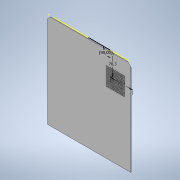
# Autodesk Inventor part: klapa
Saved by Autodesk Inventor 2020 (Build 240168000, 168)
## iProperties
Created: 2019-11-16
Part Number: klapa
Material: Ogólny
Document SubType Name: Modeling
Designer: Hubert Słomion
Density: 1 g/cm^3
Appearance: Domyślna
Author: Hubert Słomion
Autodesk Inventor part; units mm, degrees
ref_plane "YZ Plane" through (0, 0, 0) normal (1, 0, 0) x (0, 1, 0)
ref_plane "XZ Plane" through (0, 0, 0) normal (0, 1, 0) x (-1, 0, 0)
ref_plane "XY Plane" through (0, 0, 0) normal (0, 0, 1) x (1, 0, 0)
sketch "Szkic1" plane through (0, 0, 0) normal (0, 0, 1) x (1, 0, 0)
  line L0 (0, 0) -> (265, 0)
  line L1 (265, 0) -> (265, -300)
  line L2 (265, -300) -> (0, -300)
  line L3 (0, -300) -> (0, 0)
  dimension "d0" = 265
  dimension "d1" = 300
  constraints: 8 end point, 2 parallel, 1 horizontal, 1 perpendicular
  measures "d0" distance of L1.end L2.end
  measures "d1" distance of L0.end L1.end
extrude "Wyciągnięcie proste1" add sketch "Szkic1" along normal blind 4.9
chamfer "Faza2" distance 3 angle 45 4 edges at (132.5, 0, 0) (265, -150, 0) (0, -150, 0) (132.5, -300, 0)
chamfer "Faza3" distance 10 angle 45 2 edges at (1.5, -1.5, 1.5) (263.5, -1.5, 1.5)
sketch "Szkic2" plane through (0, 0, 0) normal (0, 0, -1) x (-1, 0, 0)
  line L0 (-265.2372, -89.5754) -> (-194.8372, -89.5754) construction
  line L1 (-194.8372, 0) -> (-194.8372, -139.5081) construction
  point P0 (0, 0)
  dimension "d13" = 70.4
  constraints: 4 end point, 1 horizontal, 1 vertical
  measures "d13" distance of L0.start L0.end
sketch "Szkic3" plane through (0, 0, 0) normal (0, 0, -1) x (-1, 0, 0)
  line L0 (-12.2474, 0) -> (-252.7526, 0) projected
  line L1 (-195.0449, 0) -> (-124.7449, 0)
  line L2 (-195.0449, 0) -> (-195.0449, -70.3)
  line L3 (-195.0449, 0) -> (-124.7449, 0) construction
  point P0 (0, 0)
  dimension "d15" = 70.3
  dimension "d16" = 90
  constraints: 6 end point, 2 point on line, 1 horizontal, 1 perpendicular, 1 vertical
  measures "d15" distance of L1.start L2.end
  measures "d16" angle of L2 L3
sketch "Szkic5" plane through (0, 0, 0) normal (0, 0, -1) x (-1, 0, 0)
  circle A0 centre (-245.1475, -44.0527) radius 0.875
  line L0 (-195.0449, 0) -> (-195.0449, -70.3) projected
  line L1 (-265.2372, -89.5754) -> (-194.8372, -89.5754) construction
  circle A1 centre (-245.1475, -47.0527) radius 0.875
  circle A2 centre (-245.1475, -50.0527) radius 0.875
  circle A3 centre (-245.1475, -53.0527) radius 0.875
  circle A4 centre (-245.1475, -56.0527) radius 0.875
  circle A5 centre (-245.1475, -59.0527) radius 0.875
  circle A6 centre (-245.1475, -62.0527) radius 0.875
  circle A7 centre (-245.1475, -65.0527) radius 0.875
  circle A8 centre (-245.1475, -68.0527) radius 0.875
  circle A9 centre (-245.1475, -71.0527) radius 0.875
  circle A10 centre (-245.1475, -74.0527) radius 0.875
  circle A11 centre (-245.1475, -77.0527) radius 0.875
  circle A12 centre (-245.1475, -80.0527) radius 0.875
  circle A13 centre (-245.1475, -83.0527) radius 0.875
  circle A14 centre (-245.1475, -86.0527) radius 0.875
  circle A15 centre (-245.1475, -89.0527) radius 0.875
  circle A16 centre (-245.1475, -92.0527) radius 0.875
  circle A17 centre (-245.1475, -95.0527) radius 0.875
  circle A18 centre (-245.1475, -98.0527) radius 0.875
  circle A19 centre (-245.1475, -101.0527) radius 0.875
  circle A20 centre (-242.1475, -44.0527) radius 0.875
  circle A21 centre (-242.1475, -47.0527) radius 0.875
  circle A22 centre (-242.1475, -50.0527) radius 0.875
  circle A23 centre (-242.1475, -53.0527) radius 0.875
  circle A24 centre (-242.1475, -56.0527) radius 0.875
  circle A25 centre (-242.1475, -59.0527) radius 0.875
  circle A26 centre (-242.1475, -62.0527) radius 0.875
  circle A27 centre (-242.1475, -65.0527) radius 0.875
  circle A28 centre (-242.1475, -68.0527) radius 0.875
  circle A29 centre (-242.1475, -71.0527) radius 0.875
  circle A30 centre (-242.1475, -74.0527) radius 0.875
  circle A31 centre (-242.1475, -77.0527) radius 0.875
  circle A32 centre (-242.1475, -80.0527) radius 0.875
  circle A33 centre (-242.1475, -83.0527) radius 0.875
  circle A34 centre (-242.1475, -86.0527) radius 0.875
  circle A35 centre (-242.1475, -89.0527) radius 0.875
  circle A36 centre (-242.1475, -92.0527) radius 0.875
  circle A37 centre (-242.1475, -95.0527) radius 0.875
  circle A38 centre (-242.1475, -98.0527) radius 0.875
  circle A39 centre (-242.1475, -101.0527) radius 0.875
  circle A40 centre (-239.1475, -44.0527) radius 0.875
  circle A41 centre (-239.1475, -47.0527) radius 0.875
  circle A42 centre (-239.1475, -50.0527) radius 0.875
  circle A43 centre (-239.1475, -53.0527) radius 0.875
  circle A44 centre (-239.1475, -56.0527) radius 0.875
  circle A45 centre (-239.1475, -59.0527) radius 0.875
  circle A46 centre (-239.1475, -62.0527) radius 0.875
  circle A47 centre (-239.1475, -65.0527) radius 0.875
  circle A48 centre (-239.1475, -68.0527) radius 0.875
  circle A49 centre (-239.1475, -71.0527) radius 0.875
  circle A50 centre (-239.1475, -74.0527) radius 0.875
  circle A51 centre (-239.1475, -77.0527) radius 0.875
  circle A52 centre (-239.1475, -80.0527) radius 0.875
  circle A53 centre (-239.1475, -83.0527) radius 0.875
  circle A54 centre (-239.1475, -86.0527) radius 0.875
  circle A55 centre (-239.1475, -89.0527) radius 0.875
  circle A56 centre (-239.1475, -92.0527) radius 0.875
  circle A57 centre (-239.1475, -95.0527) radius 0.875
  circle A58 centre (-239.1475, -98.0527) radius 0.875
  circle A59 centre (-239.1475, -101.0527) radius 0.875
  circle A60 centre (-236.1475, -44.0527) radius 0.875
  circle A61 centre (-236.1475, -47.0527) radius 0.875
  circle A62 centre (-236.1475, -50.0527) radius 0.875
  circle A63 centre (-236.1475, -53.0527) radius 0.875
  circle A64 centre (-236.1475, -56.0527) radius 0.875
  circle A65 centre (-236.1475, -59.0527) radius 0.875
  circle A66 centre (-236.1475, -62.0527) radius 0.875
  circle A67 centre (-236.1475, -65.0527) radius 0.875
  circle A68 centre (-236.1475, -68.0527) radius 0.875
  circle A69 centre (-236.1475, -71.0527) radius 0.875
  circle A70 centre (-236.1475, -74.0527) radius 0.875
  circle A71 centre (-236.1475, -77.0527) radius 0.875
  circle A72 centre (-236.1475, -80.0527) radius 0.875
  circle A73 centre (-236.1475, -83.0527) radius 0.875
  circle A74 centre (-236.1475, -86.0527) radius 0.875
  circle A75 centre (-236.1475, -89.0527) radius 0.875
  circle A76 centre (-236.1475, -92.0527) radius 0.875
  circle A77 centre (-236.1475, -95.0527) radius 0.875
  circle A78 centre (-236.1475, -98.0527) radius 0.875
  circle A79 centre (-236.1475, -101.0527) radius 0.875
  circle A80 centre (-233.1475, -44.0527) radius 0.875
  circle A81 centre (-233.1475, -47.0527) radius 0.875
  circle A82 centre (-233.1475, -50.0527) radius 0.875
  circle A83 centre (-233.1475, -53.0527) radius 0.875
  circle A84 centre (-233.1475, -56.0527) radius 0.875
  circle A85 centre (-233.1475, -59.0527) radius 0.875
  circle A86 centre (-233.1475, -62.0527) radius 0.875
  circle A87 centre (-233.1475, -65.0527) radius 0.875
  circle A88 centre (-233.1475, -68.0527) radius 0.875
  circle A89 centre (-233.1475, -71.0527) radius 0.875
  circle A90 centre (-233.1475, -74.0527) radius 0.875
  circle A91 centre (-233.1475, -77.0527) radius 0.875
  circle A92 centre (-233.1475, -80.0527) radius 0.875
  circle A93 centre (-233.1475, -83.0527) radius 0.875
  circle A94 centre (-233.1475, -86.0527) radius 0.875
  circle A95 centre (-233.1475, -89.0527) radius 0.875
  circle A96 centre (-233.1475, -92.0527) radius 0.875
  circle A97 centre (-233.1475, -95.0527) radius 0.875
  circle A98 centre (-233.1475, -98.0527) radius 0.875
  circle A99 centre (-233.1475, -101.0527) radius 0.875
  circle A100 centre (-230.1475, -44.0527) radius 0.875
  circle A101 centre (-230.1475, -47.0527) radius 0.875
  circle A102 centre (-230.1475, -50.0527) radius 0.875
  circle A103 centre (-230.1475, -53.0527) radius 0.875
  circle A104 centre (-230.1475, -56.0527) radius 0.875
  circle A105 centre (-230.1475, -59.0527) radius 0.875
  circle A106 centre (-230.1475, -62.0527) radius 0.875
  circle A107 centre (-230.1475, -65.0527) radius 0.875
  circle A108 centre (-230.1475, -68.0527) radius 0.875
  circle A109 centre (-230.1475, -71.0527) radius 0.875
  circle A110 centre (-230.1475, -74.0527) radius 0.875
  circle A111 centre (-230.1475, -77.0527) radius 0.875
  circle A112 centre (-230.1475, -80.0527) radius 0.875
  circle A113 centre (-230.1475, -83.0527) radius 0.875
  circle A114 centre (-230.1475, -86.0527) radius 0.875
  circle A115 centre (-230.1475, -89.0527) radius 0.875
  circle A116 centre (-230.1475, -92.0527) radius 0.875
  circle A117 centre (-230.1475, -95.0527) radius 0.875
  circle A118 centre (-230.1475, -98.0527) radius 0.875
  circle A119 centre (-230.1475, -101.0527) radius 0.875
  circle A120 centre (-227.1475, -44.0527) radius 0.875
  circle A121 centre (-227.1475, -47.0527) radius 0.875
  circle A122 centre (-227.1475, -50.0527) radius 0.875
  circle A123 centre (-227.1475, -53.0527) radius 0.875
  circle A124 centre (-227.1475, -56.0527) radius 0.875
  circle A125 centre (-227.1475, -59.0527) radius 0.875
  circle A126 centre (-227.1475, -62.0527) radius 0.875
  circle A127 centre (-227.1475, -65.0527) radius 0.875
  circle A128 centre (-227.1475, -68.0527) radius 0.875
  circle A129 centre (-227.1475, -71.0527) radius 0.875
  circle A130 centre (-227.1475, -74.0527) radius 0.875
  circle A131 centre (-227.1475, -77.0527) radius 0.875
  circle A132 centre (-227.1475, -80.0527) radius 0.875
  circle A133 centre (-227.1475, -83.0527) radius 0.875
  circle A134 centre (-227.1475, -86.0527) radius 0.875
  circle A135 centre (-227.1475, -89.0527) radius 0.875
  circle A136 centre (-227.1475, -92.0527) radius 0.875
  circle A137 centre (-227.1475, -95.0527) radius 0.875
  circle A138 centre (-227.1475, -98.0527) radius 0.875
  circle A139 centre (-227.1475, -101.0527) radius 0.875
  circle A140 centre (-224.1475, -44.0527) radius 0.875
  circle A141 centre (-224.1475, -47.0527) radius 0.875
  circle A142 centre (-224.1475, -50.0527) radius 0.875
  circle A143 centre (-224.1475, -53.0527) radius 0.875
  circle A144 centre (-224.1475, -56.0527) radius 0.875
  circle A145 centre (-224.1475, -59.0527) radius 0.875
  circle A146 centre (-224.1475, -62.0527) radius 0.875
  circle A147 centre (-224.1475, -65.0527) radius 0.875
  circle A148 centre (-224.1475, -68.0527) radius 0.875
  circle A149 centre (-224.1475, -71.0527) radius 0.875
  circle A150 centre (-224.1475, -74.0527) radius 0.875
  circle A151 centre (-224.1475, -77.0527) radius 0.875
  circle A152 centre (-224.1475, -80.0527) radius 0.875
  circle A153 centre (-224.1475, -83.0527) radius 0.875
  circle A154 centre (-224.1475, -86.0527) radius 0.875
  circle A155 centre (-224.1475, -89.0527) radius 0.875
  circle A156 centre (-224.1475, -92.0527) radius 0.875
  circle A157 centre (-224.1475, -95.0527) radius 0.875
  circle A158 centre (-224.1475, -98.0527) radius 0.875
  circle A159 centre (-224.1475, -101.0527) radius 0.875
  circle A160 centre (-221.1475, -44.0527) radius 0.875
  circle A161 centre (-221.1475, -47.0527) radius 0.875
  circle A162 centre (-221.1475, -50.0527) radius 0.875
  circle A163 centre (-221.1475, -53.0527) radius 0.875
  circle A164 centre (-221.1475, -56.0527) radius 0.875
  circle A165 centre (-221.1475, -59.0527) radius 0.875
  circle A166 centre (-221.1475, -62.0527) radius 0.875
  circle A167 centre (-221.1475, -65.0527) radius 0.875
  circle A168 centre (-221.1475, -68.0527) radius 0.875
  circle A169 centre (-221.1475, -71.0527) radius 0.875
  circle A170 centre (-221.1475, -74.0527) radius 0.875
  circle A171 centre (-221.1475, -77.0527) radius 0.875
  circle A172 centre (-221.1475, -80.0527) radius 0.875
  circle A173 centre (-221.1475, -83.0527) radius 0.875
  circle A174 centre (-221.1475, -86.0527) radius 0.875
  circle A175 centre (-221.1475, -89.0527) radius 0.875
  circle A176 centre (-221.1475, -92.0527) radius 0.875
  circle A177 centre (-221.1475, -95.0527) radius 0.875
  circle A178 centre (-221.1475, -98.0527) radius 0.875
  circle A179 centre (-221.1475, -101.0527) radius 0.875
  circle A180 centre (-218.1475, -44.0527) radius 0.875
  circle A181 centre (-218.1475, -47.0527) radius 0.875
  circle A182 centre (-218.1475, -50.0527) radius 0.875
  circle A183 centre (-218.1475, -53.0527) radius 0.875
  circle A184 centre (-218.1475, -56.0527) radius 0.875
  circle A185 centre (-218.1475, -59.0527) radius 0.875
  circle A186 centre (-218.1475, -62.0527) radius 0.875
  circle A187 centre (-218.1475, -65.0527) radius 0.875
  circle A188 centre (-218.1475, -68.0527) radius 0.875
  circle A189 centre (-218.1475, -71.0527) radius 0.875
  circle A190 centre (-218.1475, -74.0527) radius 0.875
  circle A191 centre (-218.1475, -77.0527) radius 0.875
  circle A192 centre (-218.1475, -80.0527) radius 0.875
  circle A193 centre (-218.1475, -83.0527) radius 0.875
  circle A194 centre (-218.1475, -86.0527) radius 0.875
  circle A195 centre (-218.1475, -89.0527) radius 0.875
  circle A196 centre (-218.1475, -92.0527) radius 0.875
  circle A197 centre (-218.1475, -95.0527) radius 0.875
  circle A198 centre (-218.1475, -98.0527) radius 0.875
  circle A199 centre (-218.1475, -101.0527) radius 0.875
  circle A200 centre (-215.1475, -44.0527) radius 0.875
  circle A201 centre (-215.1475, -47.0527) radius 0.875
  circle A202 centre (-215.1475, -50.0527) radius 0.875
  circle A203 centre (-215.1475, -53.0527) radius 0.875
  circle A204 centre (-215.1475, -56.0527) radius 0.875
  circle A205 centre (-215.1475, -59.0527) radius 0.875
  circle A206 centre (-215.1475, -62.0527) radius 0.875
  circle A207 centre (-215.1475, -65.0527) radius 0.875
  circle A208 centre (-215.1475, -68.0527) radius 0.875
  circle A209 centre (-215.1475, -71.0527) radius 0.875
  circle A210 centre (-215.1475, -74.0527) radius 0.875
  circle A211 centre (-215.1475, -77.0527) radius 0.875
  circle A212 centre (-215.1475, -80.0527) radius 0.875
  circle A213 centre (-215.1475, -83.0527) radius 0.875
  circle A214 centre (-215.1475, -86.0527) radius 0.875
  circle A215 centre (-215.1475, -89.0527) radius 0.875
  circle A216 centre (-215.1475, -92.0527) radius 0.875
  circle A217 centre (-215.1475, -95.0527) radius 0.875
  circle A218 centre (-215.1475, -98.0527) radius 0.875
  circle A219 centre (-215.1475, -101.0527) radius 0.875
  circle A220 centre (-212.1475, -44.0527) radius 0.875
  circle A221 centre (-212.1475, -47.0527) radius 0.875
  circle A222 centre (-212.1475, -50.0527) radius 0.875
  circle A223 centre (-212.1475, -53.0527) radius 0.875
  circle A224 centre (-212.1475, -56.0527) radius 0.875
  circle A225 centre (-212.1475, -59.0527) radius 0.875
  circle A226 centre (-212.1475, -62.0527) radius 0.875
  circle A227 centre (-212.1475, -65.0527) radius 0.875
  circle A228 centre (-212.1475, -68.0527) radius 0.875
  circle A229 centre (-212.1475, -71.0527) radius 0.875
  circle A230 centre (-212.1475, -74.0527) radius 0.875
  circle A231 centre (-212.1475, -77.0527) radius 0.875
  circle A232 centre (-212.1475, -80.0527) radius 0.875
  circle A233 centre (-212.1475, -83.0527) radius 0.875
  circle A234 centre (-212.1475, -86.0527) radius 0.875
  circle A235 centre (-212.1475, -89.0527) radius 0.875
  circle A236 centre (-212.1475, -92.0527) radius 0.875
  circle A237 centre (-212.1475, -95.0527) radius 0.875
  circle A238 centre (-212.1475, -98.0527) radius 0.875
  circle A239 centre (-212.1475, -101.0527) radius 0.875
  circle A240 centre (-209.1475, -44.0527) radius 0.875
  circle A241 centre (-209.1475, -47.0527) radius 0.875
  circle A242 centre (-209.1475, -50.0527) radius 0.875
  circle A243 centre (-209.1475, -53.0527) radius 0.875
  circle A244 centre (-209.1475, -56.0527) radius 0.875
  circle A245 centre (-209.1475, -59.0527) radius 0.875
  circle A246 centre (-209.1475, -62.0527) radius 0.875
  circle A247 centre (-209.1475, -65.0527) radius 0.875
  circle A248 centre (-209.1475, -68.0527) radius 0.875
  circle A249 centre (-209.1475, -71.0527) radius 0.875
  circle A250 centre (-209.1475, -74.0527) radius 0.875
  circle A251 centre (-209.1475, -77.0527) radius 0.875
  circle A252 centre (-209.1475, -80.0527) radius 0.875
  circle A253 centre (-209.1475, -83.0527) radius 0.875
  circle A254 centre (-209.1475, -86.0527) radius 0.875
  circle A255 centre (-209.1475, -89.0527) radius 0.875
  circle A256 centre (-209.1475, -92.0527) radius 0.875
  circle A257 centre (-209.1475, -95.0527) radius 0.875
  circle A258 centre (-209.1475, -98.0527) radius 0.875
  circle A259 centre (-209.1475, -101.0527) radius 0.875
  circle A260 centre (-206.1475, -44.0527) radius 0.875
  circle A261 centre (-206.1475, -47.0527) radius 0.875
  circle A262 centre (-206.1475, -50.0527) radius 0.875
  circle A263 centre (-206.1475, -53.0527) radius 0.875
  circle A264 centre (-206.1475, -56.0527) radius 0.875
  circle A265 centre (-206.1475, -59.0527) radius 0.875
  circle A266 centre (-206.1475, -62.0527) radius 0.875
  circle A267 centre (-206.1475, -65.0527) radius 0.875
  circle A268 centre (-206.1475, -68.0527) radius 0.875
  circle A269 centre (-206.1475, -71.0527) radius 0.875
  circle A270 centre (-206.1475, -74.0527) radius 0.875
  circle A271 centre (-206.1475, -77.0527) radius 0.875
  circle A272 centre (-206.1475, -80.0527) radius 0.875
  circle A273 centre (-206.1475, -83.0527) radius 0.875
  circle A274 centre (-206.1475, -86.0527) radius 0.875
  circle A275 centre (-206.1475, -89.0527) radius 0.875
  circle A276 centre (-206.1475, -92.0527) radius 0.875
  circle A277 centre (-206.1475, -95.0527) radius 0.875
  circle A278 centre (-206.1475, -98.0527) radius 0.875
  circle A279 centre (-206.1475, -101.0527) radius 0.875
  circle A280 centre (-203.1475, -44.0527) radius 0.875
  circle A281 centre (-203.1475, -47.0527) radius 0.875
  circle A282 centre (-203.1475, -50.0527) radius 0.875
  circle A283 centre (-203.1475, -53.0527) radius 0.875
  circle A284 centre (-203.1475, -56.0527) radius 0.875
  circle A285 centre (-203.1475, -59.0527) radius 0.875
  circle A286 centre (-203.1475, -62.0527) radius 0.875
  circle A287 centre (-203.1475, -65.0527) radius 0.875
  circle A288 centre (-203.1475, -68.0527) radius 0.875
  circle A289 centre (-203.1475, -71.0527) radius 0.875
  circle A290 centre (-203.1475, -74.0527) radius 0.875
  circle A291 centre (-203.1475, -77.0527) radius 0.875
  circle A292 centre (-203.1475, -80.0527) radius 0.875
  circle A293 centre (-203.1475, -83.0527) radius 0.875
  circle A294 centre (-203.1475, -86.0527) radius 0.875
  circle A295 centre (-203.1475, -89.0527) radius 0.875
  circle A296 centre (-203.1475, -92.0527) radius 0.875
  circle A297 centre (-203.1475, -95.0527) radius 0.875
  circle A298 centre (-203.1475, -98.0527) radius 0.875
  circle A299 centre (-203.1475, -101.0527) radius 0.875
  circle A300 centre (-200.1475, -44.0527) radius 0.875
  circle A301 centre (-200.1475, -47.0527) radius 0.875
  circle A302 centre (-200.1475, -50.0527) radius 0.875
  circle A303 centre (-200.1475, -53.0527) radius 0.875
  circle A304 centre (-200.1475, -56.0527) radius 0.875
  circle A305 centre (-200.1475, -59.0527) radius 0.875
  circle A306 centre (-200.1475, -62.0527) radius 0.875
  circle A307 centre (-200.1475, -65.0527) radius 0.875
  circle A308 centre (-200.1475, -68.0527) radius 0.875
  circle A309 centre (-200.1475, -71.0527) radius 0.875
  circle A310 centre (-200.1475, -74.0527) radius 0.875
  circle A311 centre (-200.1475, -77.0527) radius 0.875
  circle A312 centre (-200.1475, -80.0527) radius 0.875
  circle A313 centre (-200.1475, -83.0527) radius 0.875
  circle A314 centre (-200.1475, -86.0527) radius 0.875
  circle A315 centre (-200.1475, -89.0527) radius 0.875
  circle A316 centre (-200.1475, -92.0527) radius 0.875
  circle A317 centre (-200.1475, -95.0527) radius 0.875
  circle A318 centre (-200.1475, -98.0527) radius 0.875
  circle A319 centre (-200.1475, -101.0527) radius 0.875
  circle A320 centre (-197.1475, -44.0527) radius 0.875
  circle A321 centre (-197.1475, -47.0527) radius 0.875
  circle A322 centre (-197.1475, -50.0527) radius 0.875
  circle A323 centre (-197.1475, -53.0527) radius 0.875
  circle A324 centre (-197.1475, -56.0527) radius 0.875
  circle A325 centre (-197.1475, -59.0527) radius 0.875
  circle A326 centre (-197.1475, -62.0527) radius 0.875
  circle A327 centre (-197.1475, -65.0527) radius 0.875
  circle A328 centre (-197.1475, -68.0527) radius 0.875
  circle A329 centre (-197.1475, -71.0527) radius 0.875
  circle A330 centre (-197.1475, -74.0527) radius 0.875
  circle A331 centre (-197.1475, -77.0527) radius 0.875
  circle A332 centre (-197.1475, -80.0527) radius 0.875
  circle A333 centre (-197.1475, -83.0527) radius 0.875
  circle A334 centre (-197.1475, -86.0527) radius 0.875
  circle A335 centre (-197.1475, -89.0527) radius 0.875
  circle A336 centre (-197.1475, -92.0527) radius 0.875
  circle A337 centre (-197.1475, -95.0527) radius 0.875
  circle A338 centre (-197.1475, -98.0527) radius 0.875
  circle A339 centre (-197.1475, -101.0527) radius 0.875
  circle A340 centre (-194.1475, -44.0527) radius 0.875
  circle A341 centre (-194.1475, -47.0527) radius 0.875
  circle A342 centre (-194.1475, -50.0527) radius 0.875
  circle A343 centre (-194.1475, -53.0527) radius 0.875
  circle A344 centre (-194.1475, -56.0527) radius 0.875
  circle A345 centre (-194.1475, -59.0527) radius 0.875
  circle A346 centre (-194.1475, -62.0527) radius 0.875
  circle A347 centre (-194.1475, -65.0527) radius 0.875
  circle A348 centre (-194.1475, -68.0527) radius 0.875
  circle A349 centre (-194.1475, -71.0527) radius 0.875
  circle A350 centre (-194.1475, -74.0527) radius 0.875
  circle A351 centre (-194.1475, -77.0527) radius 0.875
  circle A352 centre (-194.1475, -80.0527) radius 0.875
  circle A353 centre (-194.1475, -83.0527) radius 0.875
  circle A354 centre (-194.1475, -86.0527) radius 0.875
  circle A355 centre (-194.1475, -89.0527) radius 0.875
  circle A356 centre (-194.1475, -92.0527) radius 0.875
  circle A357 centre (-194.1475, -95.0527) radius 0.875
  circle A358 centre (-194.1475, -98.0527) radius 0.875
  circle A359 centre (-194.1475, -101.0527) radius 0.875
  circle A360 centre (-191.1475, -44.0527) radius 0.875
  circle A361 centre (-191.1475, -47.0527) radius 0.875
  circle A362 centre (-191.1475, -50.0527) radius 0.875
  circle A363 centre (-191.1475, -53.0527) radius 0.875
  circle A364 centre (-191.1475, -56.0527) radius 0.875
  circle A365 centre (-191.1475, -59.0527) radius 0.875
  circle A366 centre (-191.1475, -62.0527) radius 0.875
  circle A367 centre (-191.1475, -65.0527) radius 0.875
  circle A368 centre (-191.1475, -68.0527) radius 0.875
  circle A369 centre (-191.1475, -71.0527) radius 0.875
  circle A370 centre (-191.1475, -74.0527) radius 0.875
  circle A371 centre (-191.1475, -77.0527) radius 0.875
  circle A372 centre (-191.1475, -80.0527) radius 0.875
  circle A373 centre (-191.1475, -83.0527) radius 0.875
  circle A374 centre (-191.1475, -86.0527) radius 0.875
  circle A375 centre (-191.1475, -89.0527) radius 0.875
  circle A376 centre (-191.1475, -92.0527) radius 0.875
  circle A377 centre (-191.1475, -95.0527) radius 0.875
  circle A378 centre (-191.1475, -98.0527) radius 0.875
  circle A379 centre (-191.1475, -101.0527) radius 0.875
  circle A380 centre (-188.1475, -44.0527) radius 0.875
  circle A381 centre (-188.1475, -47.0527) radius 0.875
  circle A382 centre (-188.1475, -50.0527) radius 0.875
  circle A383 centre (-188.1475, -53.0527) radius 0.875
  circle A384 centre (-188.1475, -56.0527) radius 0.875
  circle A385 centre (-188.1475, -59.0527) radius 0.875
  circle A386 centre (-188.1475, -62.0527) radius 0.875
  circle A387 centre (-188.1475, -65.0527) radius 0.875
  circle A388 centre (-188.1475, -68.0527) radius 0.875
  circle A389 centre (-188.1475, -71.0527) radius 0.875
  circle A390 centre (-188.1475, -74.0527) radius 0.875
  circle A391 centre (-188.1475, -77.0527) radius 0.875
  circle A392 centre (-188.1475, -80.0527) radius 0.875
  circle A393 centre (-188.1475, -83.0527) radius 0.875
  circle A394 centre (-188.1475, -86.0527) radius 0.875
  circle A395 centre (-188.1475, -89.0527) radius 0.875
  circle A396 centre (-188.1475, -92.0527) radius 0.875
  circle A397 centre (-188.1475, -95.0527) radius 0.875
  circle A398 centre (-188.1475, -98.0527) radius 0.875
  circle A399 centre (-188.1475, -101.0527) radius 0.875
  point P0 (0, 0)
  point P1 (-242.1475, -44.0527)
  point P2 (-242.1475, -47.0527)
  point P3 (-242.1475, -50.0527)
  point P4 (-242.1475, -53.0527)
  point P5 (-242.1475, -56.0527)
  point P6 (-242.1475, -59.0527)
  point P7 (-242.1475, -62.0527)
  point P8 (-242.1475, -65.0527)
  point P9 (-242.1475, -68.0527)
  point P10 (-242.1475, -71.0527)
  point P11 (-242.1475, -74.0527)
  point P12 (-242.1475, -77.0527)
  point P13 (-242.1475, -80.0527)
  point P14 (-242.1475, -83.0527)
  point P15 (-242.1475, -86.0527)
  point P16 (-242.1475, -89.0527)
  point P17 (-242.1475, -92.0527)
  point P18 (-242.1475, -95.0527)
  point P19 (-242.1475, -98.0527)
  point P20 (-242.1475, -101.0527)
  point P21 (-239.1475, -44.0527)
  point P22 (-239.1475, -47.0527)
  point P23 (-239.1475, -50.0527)
  point P24 (-239.1475, -53.0527)
  point P25 (-239.1475, -56.0527)
  point P26 (-239.1475, -59.0527)
  point P27 (-239.1475, -62.0527)
  point P28 (-239.1475, -65.0527)
  point P29 (-239.1475, -68.0527)
  point P30 (-239.1475, -71.0527)
  point P31 (-239.1475, -74.0527)
  point P32 (-239.1475, -77.0527)
  point P33 (-239.1475, -80.0527)
  point P34 (-239.1475, -83.0527)
  point P35 (-239.1475, -86.0527)
  point P36 (-239.1475, -89.0527)
  point P37 (-239.1475, -92.0527)
  point P38 (-239.1475, -95.0527)
  point P39 (-239.1475, -98.0527)
  point P40 (-239.1475, -101.0527)
  point P41 (-236.1475, -44.0527)
  point P42 (-236.1475, -47.0527)
  point P43 (-236.1475, -50.0527)
  point P44 (-236.1475, -53.0527)
  point P45 (-236.1475, -56.0527)
  point P46 (-236.1475, -59.0527)
  point P47 (-236.1475, -62.0527)
  point P48 (-236.1475, -65.0527)
  point P49 (-236.1475, -68.0527)
  point P50 (-236.1475, -71.0527)
  point P51 (-236.1475, -74.0527)
  point P52 (-236.1475, -77.0527)
  point P53 (-236.1475, -80.0527)
  point P54 (-236.1475, -83.0527)
  point P55 (-236.1475, -86.0527)
  point P56 (-236.1475, -89.0527)
  point P57 (-236.1475, -92.0527)
  point P58 (-236.1475, -95.0527)
  point P59 (-236.1475, -98.0527)
  point P60 (-236.1475, -101.0527)
  point P61 (-233.1475, -44.0527)
  point P62 (-233.1475, -47.0527)
  point P63 (-233.1475, -50.0527)
  point P64 (-233.1475, -53.0527)
  point P65 (-233.1475, -56.0527)
  point P66 (-233.1475, -59.0527)
  point P67 (-233.1475, -62.0527)
  point P68 (-233.1475, -65.0527)
  point P69 (-233.1475, -68.0527)
  point P70 (-233.1475, -71.0527)
  point P71 (-233.1475, -74.0527)
  point P72 (-233.1475, -77.0527)
  point P73 (-233.1475, -80.0527)
  point P74 (-233.1475, -83.0527)
  point P75 (-233.1475, -86.0527)
  point P76 (-233.1475, -89.0527)
  point P77 (-233.1475, -92.0527)
  point P78 (-233.1475, -95.0527)
  point P79 (-233.1475, -98.0527)
  point P80 (-233.1475, -101.0527)
  point P81 (-230.1475, -44.0527)
  point P82 (-230.1475, -47.0527)
  point P83 (-230.1475, -50.0527)
  point P84 (-230.1475, -53.0527)
  point P85 (-230.1475, -56.0527)
  point P86 (-230.1475, -59.0527)
  point P87 (-230.1475, -62.0527)
  point P88 (-230.1475, -65.0527)
  point P89 (-230.1475, -68.0527)
  point P90 (-230.1475, -71.0527)
  point P91 (-230.1475, -74.0527)
  point P92 (-230.1475, -77.0527)
  point P93 (-230.1475, -80.0527)
  point P94 (-230.1475, -83.0527)
  point P95 (-230.1475, -86.0527)
  point P96 (-230.1475, -89.0527)
  point P97 (-230.1475, -92.0527)
  point P98 (-230.1475, -95.0527)
  point P99 (-230.1475, -98.0527)
  point P100 (-230.1475, -101.0527)
  point P101 (-227.1475, -44.0527)
  point P102 (-227.1475, -47.0527)
  point P103 (-227.1475, -50.0527)
  point P104 (-227.1475, -53.0527)
  point P105 (-227.1475, -56.0527)
  point P106 (-227.1475, -59.0527)
  point P107 (-227.1475, -62.0527)
  point P108 (-227.1475, -65.0527)
  point P109 (-227.1475, -68.0527)
  point P110 (-227.1475, -71.0527)
  point P111 (-227.1475, -74.0527)
  point P112 (-227.1475, -77.0527)
  point P113 (-227.1475, -80.0527)
  point P114 (-227.1475, -83.0527)
  point P115 (-227.1475, -86.0527)
  point P116 (-227.1475, -89.0527)
  point P117 (-227.1475, -92.0527)
  point P118 (-227.1475, -95.0527)
  point P119 (-227.1475, -98.0527)
  point P120 (-227.1475, -101.0527)
  point P121 (-224.1475, -44.0527)
  point P122 (-224.1475, -47.0527)
  point P123 (-224.1475, -50.0527)
  point P124 (-224.1475, -53.0527)
  point P125 (-224.1475, -56.0527)
  point P126 (-224.1475, -59.0527)
  point P127 (-224.1475, -62.0527)
  point P128 (-224.1475, -65.0527)
  point P129 (-224.1475, -68.0527)
  point P130 (-224.1475, -71.0527)
  point P131 (-224.1475, -74.0527)
  point P132 (-224.1475, -77.0527)
  point P133 (-224.1475, -80.0527)
  point P134 (-224.1475, -83.0527)
  point P135 (-224.1475, -86.0527)
  point P136 (-224.1475, -89.0527)
  point P137 (-224.1475, -92.0527)
  point P138 (-224.1475, -95.0527)
  point P139 (-224.1475, -98.0527)
  point P140 (-224.1475, -101.0527)
  point P141 (-221.1475, -44.0527)
  point P142 (-221.1475, -47.0527)
  point P143 (-221.1475, -50.0527)
  point P144 (-221.1475, -53.0527)
  point P145 (-221.1475, -56.0527)
  point P146 (-221.1475, -59.0527)
  point P147 (-221.1475, -62.0527)
  point P148 (-221.1475, -65.0527)
  point P149 (-221.1475, -68.0527)
  point P150 (-221.1475, -71.0527)
  point P151 (-221.1475, -74.0527)
  point P152 (-221.1475, -77.0527)
  point P153 (-221.1475, -80.0527)
  point P154 (-221.1475, -83.0527)
  point P155 (-221.1475, -86.0527)
  point P156 (-221.1475, -89.0527)
  point P157 (-221.1475, -92.0527)
  point P158 (-221.1475, -95.0527)
  point P159 (-221.1475, -98.0527)
  point P160 (-221.1475, -101.0527)
  point P161 (-218.1475, -44.0527)
  point P162 (-218.1475, -47.0527)
  point P163 (-218.1475, -50.0527)
  point P164 (-218.1475, -53.0527)
  point P165 (-218.1475, -56.0527)
  point P166 (-218.1475, -59.0527)
  point P167 (-218.1475, -62.0527)
  point P168 (-218.1475, -65.0527)
  point P169 (-218.1475, -68.0527)
  point P170 (-218.1475, -71.0527)
  point P171 (-218.1475, -74.0527)
  point P172 (-218.1475, -77.0527)
  point P173 (-218.1475, -80.0527)
  point P174 (-218.1475, -83.0527)
  point P175 (-218.1475, -86.0527)
  point P176 (-218.1475, -89.0527)
  point P177 (-218.1475, -92.0527)
  point P178 (-218.1475, -95.0527)
  point P179 (-218.1475, -98.0527)
  point P180 (-218.1475, -101.0527)
  point P181 (-215.1475, -44.0527)
  point P182 (-215.1475, -47.0527)
  point P183 (-215.1475, -50.0527)
  point P184 (-215.1475, -53.0527)
  point P185 (-215.1475, -56.0527)
  point P186 (-215.1475, -59.0527)
  point P187 (-215.1475, -62.0527)
  point P188 (-215.1475, -65.0527)
  point P189 (-215.1475, -68.0527)
  point P190 (-215.1475, -71.0527)
  point P191 (-215.1475, -74.0527)
  point P192 (-215.1475, -77.0527)
  point P193 (-215.1475, -80.0527)
  point P194 (-215.1475, -83.0527)
  point P195 (-215.1475, -86.0527)
  point P196 (-215.1475, -89.0527)
  point P197 (-215.1475, -92.0527)
  point P198 (-215.1475, -95.0527)
  point P199 (-215.1475, -98.0527)
  dimension "d30" = 1.75
  dimension "d33" = 3
  dimension "d36" = 3
  dimension "d41" = 3
  dimension "d44" = 3
  constraints: 400 centre point, 2 horizontal, 2 vertical, 1197 other
  measures "d30" diameter of A0
  measures "d33" distance of A0.centre point (-245.148, -47.053)
  measures "d36" distance of A0.centre point (-242.148, -44.053)
  measures "d41" distance of A0.centre A1.centre
  measures "d44" distance of A0.centre A20.centre
extrude "Wyciągnięcie proste4" cut sketch "Szkic5" against normal blind 119.25
